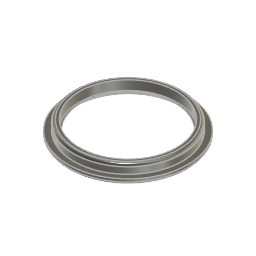
bottle_opening_adapter (Autodesk Fusion 360 design; units mm, degrees)
Autodesk Fusion 360 part; units mm, degrees
sketch "bottle_cozy" plane through (0, 0, 0) normal (0, 0, 1) x (1, 0, 0)
  circle A0 centre (0, 0) radius 29.125
  circle A1 centre (0, 0) radius 26.125
  circle A2 centre (0, 0) radius 25.25
  circle A3 centre (0, 0) radius 32.125
  dimension "d4" = 58.25
  dimension "d5" = 52.25
  dimension "d6" = 50.5
  dimension "d7" = 64.25
  constraint coincident A0.centre A1.centre
  constraint concentric A0 A1
  constraint concentric A1 A3
  measures "d4" diameter of A0
  measures "d5" diameter of A1
  measures "d6" diameter of A2
  measures "d7" diameter of A3
extrude "Extrude1" add sketch "bottle_cozy" along normal blind 3 contours A0 | A1 | A2 | A3 makes body 1
extrude "Extrude2" add sketch "bottle_cozy" along normal blind 8 contours A0 bodies 1
extrude "Extrude3" cut sketch "bottle_cozy" along normal blind 3 contours A2 bodies 1
chamfer "Chamfer1" distance 3 angle 45 1 edges at (-23.5413, -9.1308, 0) on bodies 1
fillet "Fillet1" radius 1.5 1 edges at (-29.951, -11.6169, 0) on bodies 1
fillet "Fillet2" radius 1.5 1 edges at (-27.154, -10.532, 8) on bodies 1
sketch "insert" plane through (0, 0, 0) normal (0, 0, 1) x (1, 0, 0)
  circle A0 centre (0, 0) radius 25
  circle A1 centre (0, 0) radius 28
  circle A2 centre (0, 0) radius 23.5
  dimension "d22" = 50
  dimension "d23" = 56
  dimension "d24" = 47
  constraint coincident A0.centre A1.centre
  constraint concentric A0 A2
  measures "d22" diameter of A0
  measures "d23" diameter of A1
  measures "d24" diameter of A2
extrude "Extrude4" add sketch "insert" along normal blind 6 separate body contours A0 makes body 2
extrude "Extrude5" add sketch "insert" along normal blind 3 contours A1 bodies 2
chamfer "Chamfer2" distance 3 angle 45 1 edges at (-26.1052, -10.1252, 3) on bodies 2
sketch "Sketch3" plane through (0, 0, 0) normal (0, 0, 1) x (1, 0, 0)
  circle A0 centre (0, 0) radius 25
  circle A1 centre (0, 0) radius 15
  circle A2 centre (0, 0) radius 18
  dimension "d30" = 50
  dimension "d31" = 30
  dimension "d32" = 36
  constraint coincident A0.centre A1.centre
  constraint concentric A0 A2
  measures "d30" diameter of A0
  measures "d31" diameter of A1
  measures "d32" diameter of A2
copy_body "CopyPasteBodies1" bodies 2 makes body 3
extrude "Extrude6" add sketch "Sketch3" along normal blind 3 contours A0 bodies 3
extrude "Extrude7" add sketch "Sketch3" along normal blind 30 contours A2 bodies 3
sketch "Sketch4" plane through (0, 0, 0) normal (0, 1, 0) x (1, 0, 0)
  line L0 (0, 0) -> (0, -25)
  circle A0 centre (0, -25) radius 1.5
  line L1 (0, 0) -> (0, -10)
  circle A1 centre (0, -10) radius 1.5
  line L2 (1.5, -25) -> (-1.5, -25)
  line L3 (-1.5, -25) -> (-1.5, -10)
  line L4 (-1.5, -10) -> (1.5, -10)
  line L5 (1.5, -10) -> (1.5, -25)
  dimension "d37" = 25
  dimension "d38" = 3
  dimension "d39" = 10
  dimension "d40" = 3
  dimension "d41" = 3
  dimension "d42" = 15
  constraint coincident L0.start L1.start
  constraint vertical L0
  constraint coincident L0.end A0.centre
  constraint parallel L0 L1
  constraint coincident L1.end A1.centre
  constraint horizontal L2
  constraint vertical L3
  constraint horizontal L4
  constraint vertical L5
  constraint coincident A0 L2.start
  measures "d37" distance of L0.start L0.end
  measures "d38" diameter of A0
  measures "d39" distance of L0.start L1.end
  measures "d40" diameter of A1
  measures "d41" distance of L2.start L2.end
  measures "d42" distance of L2.start L4.end
extrude "Extrude8" cut sketch "Sketch4" against normal blind 27 bodies 3
pattern_circular "C-Pattern1" count 12 over 360 about axis through (0, 0, 1.75) along (0, 0, 1) of "Extrude8"
fillet "Fillet3" radius 1.5 1 edges at (-16.7819, -6.5091, 30) on bodies 3
fillet "Fillet4" radius 1.5 1 edges at (-23.3082, -9.0404, 6) on bodies 3
fillet "Fillet5" radius 1.5 1 edges at (-23.3082, -9.0404, 6) on bodies 2
chamfer "Chamfer3" distance 1.5 angle 45 1 edges at (-13.9849, 5.4242, 0) on bodies 3
sketch "Sketch6" plane through (0, 0, 0) normal (0, 0, 1) x (1, 0, 0)
  circle A0 centre (0, 0) radius 19
  circle A1 centre (0, 0) radius 22.5
  line L0 (0, 0) -> (3, 0)
  line L1 (3, 0) -> (3, 3)
  line L2 (3, 3) -> (0, 3)
  line L3 (0, 3) -> (0, 0)
  line L4 (3, 3) -> (3, 22.2991)
  line L5 (3, 3) -> (22.2991, 3)
  line L6 (3, 3) -> (33, 3)
  line L7 (33, 3) -> (33, 33)
  line L8 (33, 33) -> (3, 33)
  line L9 (3, 33) -> (3, 3)
  dimension "d64" = 38
  dimension "d65" = 45
  dimension "d66" = 3
  dimension "d67" = 3
  dimension "d74" = 30
  dimension "d75" = 30
  constraint coincident A0.centre A1.centre
  constraint horizontal L0
  constraint vertical L1
  constraint horizontal L2
  constraint vertical L3
  constraint coincident A1 L4.end
  constraint perpendicular L2 L4
  constraint coincident A1 L5.end
  constraint perpendicular L4 L5
  constraint horizontal L6
  constraint vertical L7
  constraint horizontal L8
  constraint vertical L9
  measures "d64" diameter of A0
  measures "d65" diameter of A1
  measures "d66" distance of A0.centre L0.end
  measures "d67" distance of A0.centre L2.end
  measures "d74" distance of L1.end L6.end
  measures "d75" distance of L1.end L8.end
extrude "Extrude10" cut sketch "Sketch6" along normal blind 10 contours A0 A1 L4 L5 L6 L9 picked at (4.0622, 20.8978) bodies 3
fillet "Fillet7" radius 1.5 4 edges at (18.7617, 3, 1.5) (3, 18.7617, 1.5) (22.2991, 3, 1.5) (3, 22.2991, 1.5) on bodies 3
pattern_circular "C-Pattern3" count 4 over 360 about axis through (0, 0, 1.75) along (0, 0, 1) of "Extrude10", "Fillet7"
hidden bodies 2 3
equation "inner_dia_nescafe_classic = 64 mm"
equation "wall_thickness = 3 mm"
equation "insert_outer_dia = 50 mm"
equation "d4 = inner_dia"
equation "d5 = inner_dia - ( wall_thickness * 2 )"
equation "d6 = insert_outer_dia + 0.5 mm"
equation "d7 = inner_dia + ( wall_thickness * 2 )"
equation "d8 = wall_thickness"
equation "d10 = wall_thickness + 5 mm"
equation "d12 = wall_thickness"
equation "d14 = wall_thickness"
equation "d16 = wall_thickness / 2"
equation "d18 = wall_thickness / 2"
equation "inner_dia_nescafe_gold = 64.5 mm"
equation "inner_dia = inner_dia_jacobs"
equation "inner_dia_mason_jar = 60 mm"
equation "d22 = insert_outer_dia"
equation "d23 = insert_outer_dia + wall_thickness * 2"
equation "d24 = insert_outer_dia - wall_thickness"
equation "d25 = wall_thickness * 2"
equation "d27 = wall_thickness"
equation "d29 = wall_thickness"
equation "d30 = insert_outer_dia"
equation "d32 = 30 mm + ( wall_thickness * 2 )"
equation "d33 = wall_thickness"
equation "d64 = 30 mm + ( wall_thickness * 2 ) + 2 mm"
equation "d65 = insert_outer_dia - wall_thickness - 2 mm"
equation "inner_dia_jacobs = 58.25 mm"
named bodies: "bottle_cozy", "insert", "progration_basket_30m_closed"
